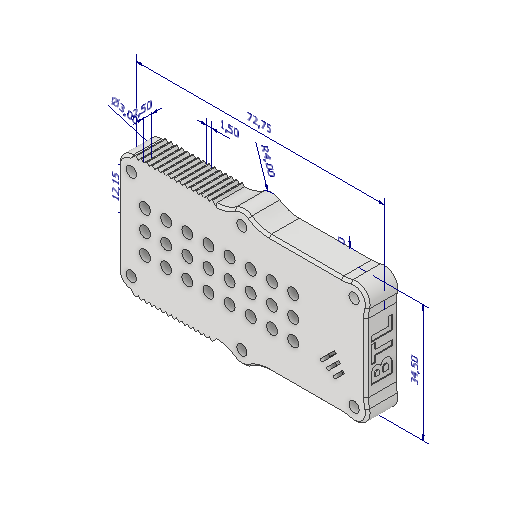
# Autodesk Inventor part: 3DP_PLA_Case_top_half
Saved by Autodesk Inventor 2025 (Build 290162010, 162A)
## iProperties
Created: 2018-09-08
Part Number: 3DP_PLA_Case_top_half
Material: ABS Plastic
Document SubType Name: Modeling
Designer: Andrzej
Density: 1.06 g/cm^3
Appearance: Smooth - White
Author: Andrzej
Autodesk Inventor part; units mm, degrees
ref_plane "YZ Plane" through (0, 0, 0) normal (1, 0, 0) x (0, 1, 0)
ref_plane "XZ Plane" through (0, 0, 0) normal (0, 1, 0) x (-1, 0, 0)
ref_plane "XY Plane" through (0, 0, 0) normal (0, 0, 1) x (1, 0, 0)
sketch "Sketch1" plane through (0, 0, 0) normal (0, 0, 1) x (1, 0, 0)
  line L0 (-37.547, 17.25) -> (35.203, 17.25)
  line L1 (35.203, 17.25) -> (35.203, -17.25)
  line L2 (35.203, -17.25) -> (-37.547, -17.25)
  line L3 (-37.547, -17.25) -> (-37.547, 17.25)
  line L4 (32.203, 14.25) -> (-34.547, 14.25)
  line L5 (-34.547, 14.25) -> (-34.547, -14.25)
  line L6 (-34.547, -14.25) -> (32.203, -14.25)
  line L7 (32.203, -14.25) -> (32.203, 14.25)
  point P0 (0, 0)
  dimension "d0" = 72.75
  dimension "d1" = 34.5
  dimension "d2" = 3
  dimension "d94" = 17.25
  constraints: 16 end point, 4 parallel, 2 perpendicular, 1 horizontal, 3 other
  measures "d0" distance of L1.end L2.end
  measures "d1" distance of L0.end L1.end
  measures "d2" distance between parallel lines of L0 L4
  measures "d94" distance from line of point (0, 0) L2
extrude "Extrusion1" add sketch "Sketch1" along normal blind 2.5 contours L0 L1 L2 L3 | L7 L6 L5 L4
extrude "Extrusion2" add sketch "Sketch1" against normal blind 6.3
fillet "Fillet1" radius 6 4 edges at (35.203, 17.25, -1.9) (32.203, 14.25, -3.15) (35.203, -17.25, -1.9) (32.203, -14.25, -3.15)
fillet "Fillet1" radius 4 4 edges at (-34.547, 14.25, -3.15) (-37.547, 17.25, -1.9) (-34.547, -14.25, -3.15) (-37.547, -17.25, -1.9)
sketch "Sketch2" plane through (0, 0, -6.3) normal (0, 0, -1) x (-1, 0, 0)
  line L0 (34.547, 10.25) -> (34.547, -10.25) projected
  arc A0 (30.547, -14.25) -> (34.547, -10.25) centre (30.547, -10.25) ccw projected
  line L1 (30.547, -14.25) -> (-26.203, -14.25) projected
  arc A1 (-32.203, -8.25) -> (-26.203, -14.25) centre (-26.203, -8.25) ccw projected
  line L2 (-32.203, -8.25) -> (-32.203, 8.25) projected
  arc A2 (-26.203, 14.25) -> (-32.203, 8.25) centre (-26.203, 8.25) ccw projected
  line L3 (-26.203, 14.25) -> (30.547, 14.25) projected
  arc A3 (34.547, 10.25) -> (30.547, 14.25) centre (30.547, 10.25) ccw projected
  arc A4 (33.547, -17.25) -> (37.547, -13.25) centre (33.547, -13.25) ccw projected
  line L4 (37.547, -13.25) -> (37.547, 13.25) projected
  arc A5 (37.547, 13.25) -> (33.547, 17.25) centre (33.547, 13.25) ccw projected
  line L5 (33.547, 17.25) -> (-29.203, 17.25) projected
  arc A6 (-29.203, 17.25) -> (-35.203, 11.25) centre (-29.203, 11.25) ccw projected
  line L6 (-35.203, 11.25) -> (-35.203, -11.25) projected
  arc A7 (-35.203, -11.25) -> (-29.203, -17.25) centre (-29.203, -11.25) ccw projected
  line L7 (-29.203, -17.25) -> (33.547, -17.25) projected
  circle A8 centre (33.547, 13.25) radius 4
  circle A9 centre (33.547, -13.25) radius 4
  circle A10 centre (1.172, -15.75) radius 4
  circle A11 centre (1.172, 15.75) radius 4
  circle A12 centre (-31.703, 13.75) radius 4
  circle A13 centre (-31.703, -13.75) radius 4
  point P0 (0, 0)
  dimension "d9" = 8
  dimension "d10" = 8
  dimension "d11" = 8
  dimension "d12" = 8
  dimension "d13" = 8
  dimension "d14" = 8
  dimension "d15" = 72.75
  dimension "d16" = 36.375
  dimension "d17" = 1.5
  dimension "d18" = 1.5
  dimension "d19" = 3.5
  dimension "d20" = 3.5
  dimension "d21" = 3.5
  constraints: 6 centre point, 2 coincident, 2 vertical alignment
  measures "d9" diameter of A8
  measures "d10" diameter of A9
  measures "d11" diameter of A10
  measures "d12" diameter of A11
  measures "d13" diameter of A12
  measures "d14" diameter of A13
  measures "d15" distance between parallel lines of L6 L4
  measures "d16" distance from line of L4 A10.centre
  measures "d17" distance from line of L5 A11.centre
  measures "d18" distance from line of L7 A10.centre
  measures "d19" distance from line of A13.centre L7
  measures "d20" distance from line of A13.centre L6
  measures "d21" distance from line of A12.centre L5
extrude "Extrusion3" add sketch "Sketch2" against normal up to surface (8.8 mm away) contours A3 L3 A8 A5 L0 | L0 A8 L3 A3 | A9 A4 L1 A0 L0 | L0 A0 L1 A9 | A11 L3 | L3 A11 L5 | A10 L7 L1 | L1 A10 | L5 A11 | A10 L7 | A12 A2 | A2 A12 A6 | A13 A7 A1 | A1 A13 | A6 A12 | A13 A7
hole "Hole1" at (31.703, -13.75, -6.3) at (-1.172, -15.75, -6.3) at (-33.547, -13.25, -6.3) at (-33.547, 13.25, -6.3) at (-1.172, 15.75, -6.3) at (31.703, 13.75, -6.3) direction (0, 0, 1) diameter 3 end through all both
sketch "Sketch3" plane through (-37.547, -13.25, 2.5) normal (-1, 0, 0) x (0, 0, 1)
  line L0 (0, 0) -> (-8.8, 0) projected
  line L1 (0, 26.5) -> (0, 0) projected
  line L2 (-8.8, 26.5) -> (0, 26.5) projected
  line L3 (-8.8, 0) -> (-8.8, 26.5) projected
  line L4 (-8.8, 5) -> (-8.8, 21.5) projected
  line L5 (-8.8, 19.325) -> (-6.1, 19.325)
  line L6 (-6.1, 19.325) -> (-6.1, 7.175)
  line L7 (-6.1, 7.175) -> (-8.8, 7.175)
  line L8 (-8.8, 7.175) -> (-8.8, 19.325)
  point P0 (-2.5, 13.25)
  dimension "d31" = 2.7
  dimension "d32" = 12.15
  dimension "d33" = 26.5
  dimension "d34" = 7.175
  constraints: 8 end point, 2 parallel, 1 horizontal, 1 perpendicular, 1 point on line
  measures "d31" distance of L6.end L7.end
  measures "d32" distance of L5.end L6.end
  measures "d33" distance between parallel lines of L0 L2
  measures "d34" distance between parallel lines of L2 L5
extrude "Extrusion4" cut sketch "Sketch3" against normal blind 8 contours L3 L5 L6 L7
sketch "Sketch4" plane through (0, 0, 0) normal (0, 0, -1) x (-1, 0, 0)
  arc A0 (34.547, -9.377) -> (29.674, -14.25) centre (33.547, -13.25) ccw projected
  line L0 (34.547, -9.377) -> (34.547, 9.377) projected
  arc A1 (29.674, 14.25) -> (34.547, 9.377) centre (33.547, 13.25) ccw projected
  line L1 (29.674, 14.25) -> (4.8801, 14.25) projected
  arc A2 (-2.5361, 14.25) -> (4.8801, 14.25) centre (1.172, 15.75) ccw projected
  line L2 (-2.5361, 14.25) -> (-26.203, 14.25) projected
  arc A3 (-26.203, 14.25) -> (-27.7148, 14.0564) centre (-26.203, 8.25) ccw projected
  arc A4 (-32.0095, 9.7618) -> (-27.7148, 14.0564) centre (-31.703, 13.75) ccw projected
  arc A5 (-32.0095, 9.7618) -> (-32.203, 8.25) centre (-26.203, 8.25) ccw projected
  line L3 (-32.203, 8.25) -> (-32.203, -8.25) projected
  arc A6 (-32.203, -8.25) -> (-32.0095, -9.7618) centre (-26.203, -8.25) ccw projected
  arc A7 (-27.7148, -14.0564) -> (-32.0095, -9.7618) centre (-31.703, -13.75) ccw projected
  arc A8 (-27.7148, -14.0564) -> (-26.203, -14.25) centre (-26.203, -8.25) ccw projected
  line L4 (-26.203, -14.25) -> (-2.5361, -14.25) projected
  arc A9 (4.8801, -14.25) -> (-2.5361, -14.25) centre (1.172, -15.75) ccw projected
  line L5 (4.8801, -14.25) -> (29.674, -14.25) projected
  line L6 (-32.203, 8.25) -> (-32.203, -8.25) projected
  line L7 (-32.203, 1) -> (-26.203, 1)
  line L8 (-26.203, 1) -> (-26.203, 5)
  line L9 (-26.203, 5) -> (-32.203, 5)
  line L10 (-32.203, 5) -> (-32.203, 1)
  line L11 (4.8801, -14.25) -> (29.674, -14.25) projected
  line L12 (17.047, -14.25) -> (12.047, -14.25)
  line L13 (12.047, -14.25) -> (12.047, -8.25)
  line L14 (12.047, -8.25) -> (17.047, -8.25)
  line L15 (17.047, -8.25) -> (17.047, -14.25)
  line L16 (-2.5361, -14.25) -> (-26.203, -14.25) projected
  line L17 (-13.953, -14.25) -> (-18.953, -14.25)
  line L18 (-18.953, -14.25) -> (-18.953, -8.25)
  line L19 (-18.953, -8.25) -> (-13.953, -8.25)
  line L20 (-13.953, -8.25) -> (-13.953, -14.25)
  line L21 (29.674, 14.25) -> (4.8801, 14.25) projected
  line L22 (15.547, 14.25) -> (10.547, 14.25)
  line L23 (10.547, 14.25) -> (10.547, 8.25)
  line L24 (10.547, 8.25) -> (15.547, 8.25)
  line L25 (15.547, 8.25) -> (15.547, 14.25)
  line L26 (-2.5361, 14.25) -> (-26.203, 14.25) projected
  line L27 (-8.953, 14.25) -> (-13.953, 14.25)
  line L28 (-13.953, 14.25) -> (-13.953, 8.25)
  line L29 (-13.953, 8.25) -> (-8.953, 8.25)
  line L30 (-8.953, 8.25) -> (-8.953, 14.25)
  point P0 (0, 0)
  dimension "d37" = 6
  dimension "d38" = 4
  dimension "d39" = 15.25
  dimension "d40" = 5
  dimension "d41" = 6
  dimension "d42" = 5
  dimension "d43" = 6
  dimension "d44" = 5
  dimension "d45" = 6
  dimension "d46" = 5
  dimension "d47" = 6
  dimension "d48" = 18.25
  dimension "d49" = 19
  dimension "d50" = 17.5
  dimension "d51" = 13.25
  constraints: 40 end point, 10 parallel, 5 horizontal, 5 perpendicular, 5 point on line
  measures "d37" distance of L9.end L8.end
  measures "d38" distance of L8.end L7.end
  measures "d39" distance between parallel lines of L7 L4
  measures "d40" distance of L13.end L14.end
  measures "d41" distance of L12.end L13.end
  measures "d42" distance of L18.end L19.end
  measures "d43" distance of L17.end L18.end
  measures "d44" distance of L24.end L23.end
  measures "d45" distance of L23.end L22.end
  measures "d46" distance of L29.end L28.end
  measures "d47" distance of L28.end L27.end
  measures "d48" distance between parallel lines of L3 L28
  measures "d49" distance between parallel lines of L0 L25
  measures "d50" distance between parallel lines of L0 L15
  measures "d51" distance between parallel lines of L3 L18
extrude "Extrusion5" add sketch "Sketch4" along normal blind 6.9 contours L5 L13 L14 L15 | L25 L24 L23 L1 | L4 L18 L19 L20 | L30 L29 L28 L2 | L3 L9 L8 L7
fillet "Fillet2" radius 2 20 edges at (-17.047, -14.25, -3.15) (-12.047, -14.25, -3.15) (13.953, -14.25, -3.15) (18.953, -14.25, -3.15) (32.203, 5, -3.15) (32.203, 1, -3.15) (8.953, 14.25, -3.15) (13.953, 14.25, -3.15) (-15.547, 14.25, -3.15) (-10.547, 14.25, -3.15) (-17.047, -8.25, -3.45) (-12.047, -8.25, -3.45) (-15.547, 8.25, -3.45) (-10.547, 8.25, -3.45) (8.953, 8.25, -3.45) (13.953, 8.25, -3.45) (13.953, -8.25, -3.45) (18.953, -8.25, -3.45) (26.203, 1, -3.45) (26.203, 5, -3.45)
chamfer "Chamfer1" distance 0.6 angle 45 5 edges at (-13.047, 14.25, -6.9) (11.453, 14.25, -6.9) (32.203, 3, -6.9) (16.453, -14.25, -6.9) (-14.547, -14.25, -6.9)
fillet "Fillet3" radius 10 8 edges at (-4.8801, 17.25, -1.9) (2.5361, 17.25, -1.9) (29.7258, 17.2272, -1.9) (35.1802, 11.7728, -1.9) (35.1802, -11.7728, -1.9) (29.7258, -17.2272, -1.9) (2.5361, -17.25, -1.9) (-4.8801, -17.25, -1.9)
sketch "Sketch5" plane through (0, 0, 0) normal (0, 0, -1) x (-1, 0, 0)
  arc A0 (10.547, 12.25) -> (8.547, 14.25) centre (8.547, 12.25) ccw projected
  line L0 (8.547, 14.25) -> (4.8801, 14.25) projected
  arc A1 (-2.5361, 14.25) -> (4.8801, 14.25) centre (1.172, 15.75) ccw projected
  line L1 (-2.5361, 14.25) -> (-6.953, 14.25) projected
  arc A2 (-6.953, 14.25) -> (-8.953, 12.25) centre (-6.953, 12.25) ccw projected
  line L2 (-8.953, 12.25) -> (-8.953, 10.25) projected
  arc A3 (-10.953, 8.25) -> (-8.953, 10.25) centre (-10.953, 10.25) ccw projected
  line L3 (-10.953, 8.25) -> (-11.953, 8.25) projected
  arc A4 (-13.953, 10.25) -> (-11.953, 8.25) centre (-11.953, 10.25) ccw projected
  line L4 (-13.953, 10.25) -> (-13.953, 12.25) projected
  arc A5 (-13.953, 12.25) -> (-15.953, 14.25) centre (-15.953, 12.25) ccw projected
  line L5 (-15.953, 14.25) -> (-26.203, 14.25) projected
  arc A6 (-26.203, 14.25) -> (-27.7148, 14.0564) centre (-26.203, 8.25) ccw projected
  arc A7 (-32.0095, 9.7618) -> (-27.7148, 14.0564) centre (-31.703, 13.75) ccw projected
  arc A8 (-32.0095, 9.7618) -> (-32.203, 8.25) centre (-26.203, 8.25) ccw projected
  line L6 (-32.203, 8.25) -> (-32.203, 7) projected
  arc A9 (-32.203, 7) -> (-30.203, 5) centre (-30.203, 7) ccw projected
  line L7 (-30.203, 5) -> (-28.203, 5) projected
  arc A10 (-28.203, 1) -> (-28.203, 5) centre (-28.203, 3) ccw projected
  line L8 (-28.203, 1) -> (-30.203, 1) projected
  arc A11 (-30.203, 1) -> (-32.203, -1) centre (-30.203, -1) ccw projected
  line L9 (-32.203, -1) -> (-32.203, -8.25) projected
  arc A12 (-32.203, -8.25) -> (-32.0095, -9.7618) centre (-26.203, -8.25) ccw projected
  arc A13 (-27.7148, -14.0564) -> (-32.0095, -9.7618) centre (-31.703, -13.75) ccw projected
  arc A14 (-27.7148, -14.0564) -> (-26.203, -14.25) centre (-26.203, -8.25) ccw projected
  line L10 (-26.203, -14.25) -> (-20.953, -14.25) projected
  arc A15 (-20.953, -14.25) -> (-18.953, -12.25) centre (-20.953, -12.25) ccw projected
  line L11 (-18.953, -12.25) -> (-18.953, -10.25) projected
  arc A16 (-16.953, -8.25) -> (-18.953, -10.25) centre (-16.953, -10.25) ccw projected
  line L12 (-16.953, -8.25) -> (-15.953, -8.25) projected
  arc A17 (-13.953, -10.25) -> (-15.953, -8.25) centre (-15.953, -10.25) ccw projected
  line L13 (-13.953, -10.25) -> (-13.953, -12.25) projected
  arc A18 (-13.953, -12.25) -> (-11.953, -14.25) centre (-11.953, -12.25) ccw projected
  line L14 (-11.953, -14.25) -> (-2.5361, -14.25) projected
  arc A19 (4.8801, -14.25) -> (-2.5361, -14.25) centre (1.172, -15.75) ccw projected
  line L15 (4.8801, -14.25) -> (10.047, -14.25) projected
  arc A20 (10.047, -14.25) -> (12.047, -12.25) centre (10.047, -12.25) ccw projected
  line L16 (12.047, -12.25) -> (12.047, -10.25) projected
  arc A21 (14.047, -8.25) -> (12.047, -10.25) centre (14.047, -10.25) ccw projected
  line L17 (14.047, -8.25) -> (15.047, -8.25) projected
  arc A22 (17.047, -10.25) -> (15.047, -8.25) centre (15.047, -10.25) ccw projected
  line L18 (17.047, -10.25) -> (17.047, -12.25) projected
  arc A23 (17.047, -12.25) -> (19.047, -14.25) centre (19.047, -12.25) ccw projected
  line L19 (19.047, -14.25) -> (29.674, -14.25) projected
  arc A24 (34.547, -9.377) -> (29.674, -14.25) centre (33.547, -13.25) ccw projected
  line L20 (34.547, -9.377) -> (34.547, 9.377) projected
  arc A25 (29.674, 14.25) -> (34.547, 9.377) centre (33.547, 13.25) ccw projected
  line L21 (29.674, 14.25) -> (17.547, 14.25) projected
  arc A26 (17.547, 14.25) -> (15.547, 12.25) centre (17.547, 12.25) ccw projected
  line L22 (15.547, 12.25) -> (15.547, 10.25) projected
  arc A27 (13.547, 8.25) -> (15.547, 10.25) centre (13.547, 10.25) ccw projected
  line L23 (13.547, 8.25) -> (12.547, 8.25) projected
  arc A28 (10.547, 10.25) -> (12.547, 8.25) centre (12.547, 10.25) ccw projected
  line L24 (10.547, 10.25) -> (10.547, 12.25) projected
  line L25 (-25.9217, -2.3862) -> (-21.6791, -6.6289)
  line L26 (-21.6791, -6.6289) -> (-22.2448, -7.1946)
  line L27 (-22.2448, -7.1946) -> (-26.4874, -2.9519)
  line L28 (-26.4874, -2.9519) -> (-25.9217, -2.3862)
  line L29 (-28.3259, -6.2046) -> (-25.4974, -9.033)
  line L30 (-25.4974, -9.033) -> (-26.0631, -9.5987)
  line L31 (-26.0631, -9.5987) -> (-28.8916, -6.7703)
  line L32 (-28.8916, -6.7703) -> (-28.3259, -6.2046)
  circle A29 centre (29.547, -6) radius 1.6
  circle A30 centre (23.347, -6) radius 1.6
  circle A31 centre (17.147, -6) radius 1.6
  circle A32 centre (10.947, -6) radius 1.6
  circle A33 centre (4.747, -6) radius 1.6
  circle A34 centre (-1.453, -6) radius 1.6
  circle A35 centre (-7.653, -6) radius 1.6
  circle A36 centre (-13.853, -6) radius 1.6
  circle A37 centre (29.547, 0) radius 1.6
  circle A38 centre (23.347, 0) radius 1.6
  circle A39 centre (17.147, 0) radius 1.6
  circle A40 centre (10.947, 0) radius 1.6
  circle A41 centre (4.747, 0) radius 1.6
  circle A42 centre (-1.453, 0) radius 1.6
  circle A43 centre (-7.653, 0) radius 1.6
  circle A44 centre (-13.853, 0) radius 1.6
  circle A45 centre (29.547, 6) radius 1.6
  circle A46 centre (23.347, 6) radius 1.6
  circle A47 centre (17.147, 6) radius 1.6
  circle A48 centre (10.947, 6) radius 1.6
  circle A49 centre (4.747, 6) radius 1.6
  circle A50 centre (-1.453, 6) radius 1.6
  circle A51 centre (-7.653, 6) radius 1.6
  circle A52 centre (-13.853, 6) radius 1.6
  line L33 (-27.1238, -4.2954) -> (-23.5883, -7.8309)
  line L34 (-23.5883, -7.8309) -> (-24.1539, -8.3966)
  line L35 (-24.1539, -8.3966) -> (-27.6895, -4.8611)
  line L36 (-27.6895, -4.8611) -> (-27.1238, -4.2954)
  point P0 (0, 0)
  dimension "d59" = 6
  dimension "d60" = 0.8
  dimension "d63" = 4
  dimension "d64" = 0.8
  dimension "d69" = 3.2
  dimension "d72" = 6.2
  dimension "d75" = 6
  dimension "d78" = 8.25
  dimension "d79" = 5
  dimension "d98" = 5
  dimension "d99" = 0.8
  dimension "d100" = 0.5
  dimension "d101" = 0.5
  dimension "d102" = 1.4
  dimension "d103" = 1.4
  constraints: 24 centre point, 24 end point, 6 parallel, 3 perpendicular, 1 horizontal, 1 vertical, 46 other
  measures "d59" distance of L26.end L27.end
  measures "d60" distance of L25.end L26.end
  measures "d63" distance of L31.start L32.start
  measures "d64" distance of L29.end L31.start
  measures "d69" diameter of A29
  measures "d72" distance of A29.centre A30.centre
  measures "d75" distance of A29.centre A37.centre
  measures "d78" distance from line of L19 A29.centre
  measures "d79" distance from line of L20 A29.centre
  measures "d98" distance of L34.end L35.end
  measures "d99" distance of L34.start L34.end
  measures "d100" distance between parallel lines of L36 L28
  measures "d101" distance between parallel lines of L34 L30
  measures "d102" distance between parallel lines of L27 L33
  measures "d103" distance between parallel lines of L29 L35
extrude "Extrusion6" cut sketch "Sketch5" against normal blind 8 contours L25 L26 L27 L28 | L29 L30 L31 L32 | A29 | A30 | A31 | A32 | A33 | A34 | A35 | A36 | A37 | A38 | A39 | A40 | A41 | A42 | A43 | A44 | A45 | A46 | A47 | A48 | A49 | A50 | A51 | A52 | L33 L34 L35 L36
fillet "Fillet4" radius 2 12 edges at (-34.547, -9.377, -3.15) (-29.674, -14.25, -3.15) (-4.8801, -14.25, -3.15) (2.5361, -14.25, -3.15) (27.7148, -14.0564, -3.15) (32.0095, -9.7618, -3.15) (32.0095, 9.7618, -3.15) (27.7148, 14.0564, -3.15) (2.5361, 14.25, -3.15) (-4.8801, 14.25, -3.15) (-34.547, 9.377, -3.15) (-29.674, 14.25, -3.15)
sketch "Sketch6" plane through (0, 0, -6.3) normal (0, 0, -1) x (-1, 0, 0)
  arc A0 (3.4532, 19.0357) -> (9.1563, 17.25) centre (9.1563, 27.25) ccw projected
  line L0 (9.1563, 17.25) -> (9.9063, 18)
  line L1 (9.1563, 17.25) -> (10.6563, 17.25) construction
  line L2 (10.6563, 17.25) -> (9.9063, 18)
  line L3 (10.6563, 17.25) -> (20.7753, 17.25) construction
  line L4 (9.1563, 17.25) -> (10.6563, 17.25)
  line L5 (33.547, 17.25) -> (9.1563, 17.25) projected
  point P0 (0, 0)
  dimension "d84" = 45
  dimension "d86" = 135
  dimension "d87" = 1.5
  constraints: 10 end point, 2 horizontal, 1 collinear
  measures "d84" angle of L1 L0
  measures "d86" angle of L3 L2
  measures "d87" distance of L0.start L1.end
extrude "Extrusion7" add sketch "Sketch6" against normal up to surface (8.8 mm away)
fillet "Fillet5" radius 0.2 1 edges at (-9.9063, 18, -1.9)
pattern_linear "Rectangular Pattern1" count 15 spacing 1.6 along (-1, 0, 0) of "Extrusion7", "Fillet5"
mirror "Mirror1" about plane through (0, 0, 0) normal (0, 1, 0) of "Extrusion7", "Fillet5", "Rectangular Pattern1"
chamfer "Chamfer2" distance 0.7 angle 45 20 edges at (-36.3754, -16.0784, 2.5) (-37.547, 0, 2.5) (-36.3754, 16.0784, 2.5) (-33.3017, 17.25, 2.5) (-33.3017, -17.25, 2.5) (17.4037, -17.25, 2.5) (29.3312, -17.3397, 2.5) (34.5315, -16.5784, 2.5) (35.2927, -11.3782, 2.5) (35.203, 0, 2.5) (35.2927, 11.3782, 2.5) (34.5315, 16.5784, 2.5) (29.3312, 17.3397, 2.5) (17.4037, 17.25, 2.5) (3.8243, 17.7069, 2.5) (-1.172, 19.75, 2.5) (-6.1683, 17.7069, 2.5) (3.8243, -17.7069, 2.5) (-1.172, -19.75, 2.5) (-6.1683, -17.7069, 2.5)
sketch "Sketch7" plane through (35.203, -10.0419, -6.3) normal (1, 0, 0) x (0, 0, -1)
  line L0 (-8.1, 0) -> (-8.1, 20.0838) projected
  line L1 (0, 0) -> (-8.1, 0) projected
  line L2 (0, 20.0838) -> (0, 0) projected
  line L3 (-8.1, 20.0838) -> (0, 20.0838) projected
  line L4 (-7.1997, 2.1091) -> (-7.1997, 8.241) construction
  line L5 (-7.1997, 8.241) -> (10.7816, 8.241) construction
  line L6 (10.7816, 8.241) -> (10.7816, 2.1091) construction
  line L7 (10.7816, 2.1091) -> (-7.1997, 2.1091) construction
  spline S0 degree 2 poles (-2.9682, 7.6159) (-2.5135, 7.6159) (-1.8264, 7.2699) (-1.599, 6.9832) knots 0 0 0 1 2 2 2
  spline S1 degree 2 poles (-1.599, 6.9832) (-1.3271, 6.6371) (-1.0997, 5.8166) (-1.0997, 5.1789) knots 0 0 0 1 2 2 2
  line L8 (-1.0997, 5.1789) -> (-1.0997, 2.7418)
  line L9 (-1.0997, 2.7418) -> (-7.1997, 2.7418)
  line L10 (-7.1997, 2.7418) -> (-7.1997, 4.8922)
  spline S2 degree 2 poles (-7.1997, 4.8922) (-7.1997, 5.5645) (-7.0959, 6.2565) (-6.9328, 6.5581) knots 0 0 0 1 2 2 2
  spline S3 degree 2 poles (-6.9328, 6.5581) (-6.7597, 6.8893) (-6.1665, 7.2106) (-5.781, 7.2106) knots 0 0 0 1 2 2 2
  spline S4 degree 2 poles (-5.781, 7.2106) (-5.3361, 7.2106) (-4.6391, 6.7657) (-4.4759, 6.3702) knots 0 0 0 1 2 2 2
  line L11 (-4.4759, 6.3702) -> (-4.4463, 6.3702)
  spline S5 degree 2 poles (-4.4463, 6.3702) (-4.3276, 6.9387) (-3.5911, 7.6159) (-2.9682, 7.6159) knots 0 0 0 1 2 2 2
  spline S6 degree 2 poles (-2.993, 6.0341) (-3.2797, 6.0341) (-3.601, 5.8067) (-3.685, 5.5793) knots 0 0 0 1 2 2 2
  spline S7 degree 2 poles (-3.685, 5.5793) (-3.7394, 5.4409) (-3.7493, 4.9515) (-3.7493, 4.5461) knots 0 0 0 1 2 2 2
  line L12 (-3.7493, 4.5461) -> (-3.7493, 4.2644)
  line L13 (-3.7493, 4.2644) -> (-2.2119, 4.2644)
  line L14 (-2.2119, 4.2644) -> (-2.2119, 4.3484)
  spline S8 degree 2 poles (-2.2119, 4.3484) (-2.2119, 4.9416) (-2.2268, 5.3964) (-2.3306, 5.6337) knots 0 0 0 1 2 2 2
  spline S9 degree 2 poles (-2.3306, 5.6337) (-2.4245, 5.8413) (-2.7705, 6.0341) (-2.993, 6.0341) knots 0 0 0 1 2 2 2
  spline S10 degree 2 poles (-5.4794, 5.6534) (-5.6277, 5.6534) (-5.9392, 5.5002) (-6.0084, 5.342) knots 0 0 0 1 2 2 2
  spline S11 degree 2 poles (-6.0084, 5.342) (-6.0776, 5.1937) (-6.0875, 4.7785) (-6.0875, 4.3682) knots 0 0 0 1 2 2 2
  line L15 (-6.0875, 4.3682) -> (-6.0875, 4.2644)
  line L16 (-6.0875, 4.2644) -> (-4.7923, 4.2644)
  line L17 (-4.7923, 4.2644) -> (-4.7923, 4.4572)
  spline S12 degree 2 poles (-4.7923, 4.4572) (-4.7923, 4.8477) (-4.8071, 5.164) (-4.8862, 5.3321) knots 0 0 0 1 2 2 2
  spline S13 degree 2 poles (-4.8862, 5.3321) (-4.9752, 5.515) (-5.2768, 5.6534) (-5.4794, 5.6534) knots 0 0 0 1 2 2 2
  line L18 (-1.0997, 9.6674) -> (-6.038, 9.6674)
  line L19 (-6.038, 9.6674) -> (-6.038, 7.8631)
  line L20 (-6.038, 7.8631) -> (-7.1997, 7.8631)
  line L21 (-7.1997, 7.8631) -> (-7.1997, 13.0041)
  line L22 (-7.1997, 13.0041) -> (-6.038, 13.0041)
  line L23 (-6.038, 13.0041) -> (-6.038, 11.1998)
  line L24 (-6.038, 11.1998) -> (-1.0997, 11.1998)
  line L25 (-1.0997, 11.1998) -> (-1.0997, 9.6674)
  line L26 (-1.0997, 17.7002) -> (-1.0997, 13.6319)
  line L27 (-1.0997, 13.6319) -> (-7.1997, 13.6319)
  line L28 (-7.1997, 13.6319) -> (-7.1997, 15.1643)
  line L29 (-7.1997, 15.1643) -> (-2.2614, 15.1643)
  line L30 (-2.2614, 15.1643) -> (-2.2614, 17.7002)
  line L31 (-2.2614, 17.7002) -> (-1.0997, 17.7002)
  point P0 (-6.3, 10.0419)
  constraints: 2 other
extrude "Extrusion8" cut sketch "Sketch7" against normal blind 0.25 contours S0 S1 L8 L9 L10 S2 S3 S4 L11 S5 | L18 L19 L20 L21 L22 L23 L24 L25 | L26 L27 L28 L29 L30 L31
sketch "Sketch8" plane through (6.8124, -17.25, -6.3) normal (0, -1, 0) x (1, 0, 0)
  line L0 (0, 8.1) -> (21.1825, 8.1) projected
  line L1 (0, 0) -> (0, 8.1) projected
  line L2 (21.1825, 0) -> (0, 0) projected
  line L3 (21.1825, 8.1) -> (21.1825, 0) projected
  line L4 (2.5381, 7.0964) -> (22.7439, 7.0964) construction
  line L5 (22.7439, 7.0964) -> (22.7439, -4.5758) construction
  line L6 (22.7439, -4.5758) -> (2.5381, -4.5758) construction
  line L7 (2.5381, -4.5758) -> (2.5381, 7.0964) construction
  line L8 (8.8062, 0.9964) -> (6.9426, 0.9964)
  line L9 (6.9426, 0.9964) -> (5.2471, 3.2357)
  line L10 (5.2471, 3.2357) -> (4.6934, 3.2357)
  line L11 (4.6934, 3.2357) -> (4.6934, 0.9964)
  line L12 (4.6934, 0.9964) -> (3.1709, 0.9964)
  line L13 (3.1709, 0.9964) -> (3.1709, 7.0964)
  line L14 (3.1709, 7.0964) -> (5.6227, 7.0964)
  spline S0 degree 2 poles (5.6227, 7.0964) (6.1319, 7.0964) (6.8833, 6.9679) (7.2046, 6.7701) knots 0 0 0 1 2 2 2
  spline S1 degree 2 poles (7.2046, 6.7701) (7.5308, 6.5625) (7.9164, 5.9149) (7.9164, 5.4206) knots 0 0 0 1 2 2 2
  spline S2 degree 2 poles (7.9164, 5.4206) (7.9164, 4.7236) (7.2837, 3.8487) (6.7548, 3.5916) knots 0 0 0 1 2 2 2
  line L15 (6.7548, 3.5916) -> (8.8062, 0.9964)
  spline S3 degree 2 poles (6.3445, 5.2278) (6.3445, 5.4602) (6.1665, 5.7914) (5.9638, 5.8803) knots 0 0 0 1 2 2 2
  spline S4 degree 2 poles (5.9638, 5.8803) (5.8205, 5.9397) (5.4695, 5.9743) (5.2075, 5.9743) knots 0 0 0 1 2 2 2
  line L16 (5.2075, 5.9743) -> (4.6934, 5.9743)
  line L17 (4.6934, 5.9743) -> (4.6934, 4.3331)
  line L18 (4.6934, 4.3331) -> (5.1334, 4.3331)
  spline S5 degree 2 poles (5.1334, 4.3331) (5.4497, 4.3331) (5.8996, 4.4122) (6.0528, 4.5358) knots 0 0 0 1 2 2 2
  spline S6 degree 2 poles (6.0528, 4.5358) (6.2011, 4.6544) (6.3445, 4.9708) (6.3445, 5.2278) knots 0 0 0 1 2 2 2
  line L19 (10.4325, 0.9964) -> (10.4325, 5.9347)
  line L20 (10.4325, 5.9347) -> (8.6283, 5.9347)
  line L21 (8.6283, 5.9347) -> (8.6283, 7.0964)
  line L22 (8.6283, 7.0964) -> (13.7693, 7.0964)
  line L23 (13.7693, 7.0964) -> (13.7693, 5.9347)
  line L24 (13.7693, 5.9347) -> (11.965, 5.9347)
  line L25 (11.965, 5.9347) -> (11.965, 0.9964)
  line L26 (11.965, 0.9964) -> (10.4325, 0.9964)
  line L27 (18.4654, 0.9964) -> (14.3971, 0.9964)
  line L28 (14.3971, 0.9964) -> (14.3971, 7.0964)
  line L29 (14.3971, 7.0964) -> (15.9295, 7.0964)
  line L30 (15.9295, 7.0964) -> (15.9295, 2.1581)
  line L31 (15.9295, 2.1581) -> (18.4654, 2.1581)
  line L32 (18.4654, 2.1581) -> (18.4654, 0.9964)
  point P0 (-6.8124, 6.3)
  constraints: 2 other
extrude "Extrusion9" cut sketch "Sketch8" against normal blind 0.25 contours L8 L9 L10 L11 L12 L13 L14 S0 S1 S2 L15 | L19 L20 L21 L22 L23 L24 L25 L26 | L27 L28 L29 L30 L31 L32
sketch "Sketch9" plane through (0, 0, -6.9) normal (0, 0, -1) x (-1, 0, 0)
  arc A0 (32.1649, -17.8586) -> (32.4478, -17.8586) centre (32.3063, -17.7172) ccw projected
  line L0 (33.0563, -17.25) -> (32.4478, -17.8586) projected
  line L1 (33.0563, -17.25) -> (33.547, -17.25) projected
  arc A1 (33.547, -17.25) -> (37.547, -13.25) centre (33.547, -13.25) ccw projected
  line L2 (37.547, -13.25) -> (37.547, -6.075) projected
  line L3 (37.547, -6.075) -> (34.547, -6.075) projected
  line L4 (34.547, -6.075) -> (34.547, -7.3339) projected
  arc A2 (32.8803, -9.3059) -> (34.547, -7.3339) centre (32.547, -7.3339) ccw projected
  arc A3 (32.8803, -9.3059) -> (29.6029, -12.5833) centre (33.547, -13.25) ccw projected
  arc A4 (27.6309, -14.25) -> (29.6029, -12.5833) centre (27.6309, -12.25) ccw projected
  line L5 (27.6309, -14.25) -> (19.047, -14.25) projected
  arc A5 (17.047, -12.25) -> (19.047, -14.25) centre (19.047, -12.25) ccw projected
  line L6 (17.047, -14.25) -> (17.047, -12.25) projected
  line L7 (17.047, -14.25) -> (12.047, -14.25) projected
  line L8 (12.047, -12.25) -> (12.047, -14.25) projected
  arc A6 (10.047, -14.25) -> (12.047, -12.25) centre (10.047, -12.25) ccw projected
  line L9 (10.047, -14.25) -> (6.0454, -14.25) projected
  arc A7 (4.4209, -13.4167) -> (6.0454, -14.25) centre (6.0454, -12.25) ccw projected
  arc A8 (4.4209, -13.4167) -> (-2.077, -13.4167) centre (1.172, -15.75) ccw projected
  arc A9 (-3.7014, -14.25) -> (-2.077, -13.4167) centre (-3.7014, -12.25) ccw projected
  line L10 (-3.7014, -14.25) -> (-11.953, -14.25) projected
  arc A10 (-13.953, -12.25) -> (-11.953, -14.25) centre (-11.953, -12.25) ccw projected
  line L11 (-13.953, -14.25) -> (-13.953, -12.25) projected
  line L12 (-13.953, -14.25) -> (-18.953, -14.25) projected
  line L13 (-18.953, -12.25) -> (-18.953, -14.25) projected
  arc A11 (-20.953, -14.25) -> (-18.953, -12.25) centre (-20.953, -12.25) ccw projected
  line L14 (-20.953, -14.25) -> (-25.8935, -14.25) projected
  arc A12 (-27.83, -12.75) -> (-25.8935, -14.25) centre (-25.8935, -12.25) ccw projected
  arc A13 (-27.83, -12.75) -> (-30.703, -9.877) centre (-31.703, -13.75) ccw projected
  arc A14 (-32.203, -7.9405) -> (-30.703, -9.877) centre (-30.203, -7.9405) ccw projected
  line L15 (-32.203, -7.9405) -> (-32.203, -1) projected
  arc A15 (-30.203, 1) -> (-32.203, -1) centre (-30.203, -1) ccw projected
  line L16 (-32.203, 1) -> (-30.203, 1) projected
  line L17 (-32.203, 1) -> (-32.203, 5) projected
  line L18 (-30.203, 5) -> (-32.203, 5) projected
  arc A16 (-32.203, 7) -> (-30.203, 5) centre (-30.203, 7) ccw projected
  line L19 (-32.203, 7) -> (-32.203, 7.9405) projected
  arc A17 (-30.703, 9.877) -> (-32.203, 7.9405) centre (-30.203, 7.9405) ccw projected
  arc A18 (-30.703, 9.877) -> (-27.83, 12.75) centre (-31.703, 13.75) ccw projected
  arc A19 (-25.8935, 14.25) -> (-27.83, 12.75) centre (-25.8935, 12.25) ccw projected
  line L20 (-25.8935, 14.25) -> (-15.953, 14.25) projected
  arc A20 (-13.953, 12.25) -> (-15.953, 14.25) centre (-15.953, 12.25) ccw projected
  line L21 (-13.953, 14.25) -> (-13.953, 12.25) projected
  line L22 (-13.953, 14.25) -> (-8.953, 14.25) projected
  line L23 (-8.953, 12.25) -> (-8.953, 14.25) projected
  arc A21 (-6.953, 14.25) -> (-8.953, 12.25) centre (-6.953, 12.25) ccw projected
  line L24 (-6.953, 14.25) -> (-3.7014, 14.25) projected
  arc A22 (-2.077, 13.4167) -> (-3.7014, 14.25) centre (-3.7014, 12.25) ccw projected
  arc A23 (-2.077, 13.4167) -> (4.4209, 13.4167) centre (1.172, 15.75) ccw projected
  arc A24 (6.0454, 14.25) -> (4.4209, 13.4167) centre (6.0454, 12.25) ccw projected
  line L25 (6.0454, 14.25) -> (8.547, 14.25) projected
  arc A25 (10.547, 12.25) -> (8.547, 14.25) centre (8.547, 12.25) ccw projected
  line L26 (10.547, 14.25) -> (10.547, 12.25) projected
  line L27 (10.547, 14.25) -> (15.547, 14.25) projected
  line L28 (15.547, 12.25) -> (15.547, 14.25) projected
  arc A26 (17.547, 14.25) -> (15.547, 12.25) centre (17.547, 12.25) ccw projected
  line L29 (17.547, 14.25) -> (27.6309, 14.25) projected
  arc A27 (29.6029, 12.5833) -> (27.6309, 14.25) centre (27.6309, 12.25) ccw projected
  arc A28 (29.6029, 12.5833) -> (32.8803, 9.3059) centre (33.547, 13.25) ccw projected
  arc A29 (34.547, 7.3339) -> (32.8803, 9.3059) centre (32.547, 7.3339) ccw projected
  line L30 (34.547, 7.3339) -> (34.547, 6.075) projected
  line L31 (34.547, 6.075) -> (37.547, 6.075) projected
  line L32 (37.547, 6.075) -> (37.547, 13.25) projected
  arc A30 (37.547, 13.25) -> (33.547, 17.25) centre (33.547, 13.25) ccw projected
  line L33 (33.547, 17.25) -> (33.0563, 17.25) projected
  line L34 (33.0563, 17.25) -> (32.4478, 17.8586) projected
  arc A31 (32.4478, 17.8586) -> (32.1649, 17.8586) centre (32.3063, 17.7172) ccw projected
  line L35 (32.1649, 17.8586) -> (31.5563, 17.25) projected
  line L36 (31.5563, 17.25) -> (31.4563, 17.25) projected
  line L37 (31.4563, 17.25) -> (30.8478, 17.8586) projected
  arc A32 (30.8478, 17.8586) -> (30.5649, 17.8586) centre (30.7063, 17.7172) ccw projected
  line L38 (30.5649, 17.8586) -> (29.9563, 17.25) projected
  line L39 (29.9563, 17.25) -> (29.8563, 17.25) projected
  line L40 (29.8563, 17.25) -> (29.2478, 17.8586) projected
  arc A33 (29.2478, 17.8586) -> (28.9649, 17.8586) centre (29.1063, 17.7172) ccw projected
  line L41 (28.9649, 17.8586) -> (28.3563, 17.25) projected
  line L42 (28.3563, 17.25) -> (28.2563, 17.25) projected
  line L43 (28.2563, 17.25) -> (27.6478, 17.8586) projected
  arc A34 (27.6478, 17.8586) -> (27.3649, 17.8586) centre (27.5063, 17.7172) ccw projected
  line L44 (27.3649, 17.8586) -> (26.7563, 17.25) projected
  line L45 (26.7563, 17.25) -> (26.6563, 17.25) projected
  line L46 (26.6563, 17.25) -> (26.0478, 17.8586) projected
  arc A35 (26.0478, 17.8586) -> (25.7649, 17.8586) centre (25.9063, 17.7172) ccw projected
  line L47 (25.7649, 17.8586) -> (25.1563, 17.25) projected
  line L48 (25.1563, 17.25) -> (25.0563, 17.25) projected
  line L49 (25.0563, 17.25) -> (24.4478, 17.8586) projected
  arc A36 (24.4478, 17.8586) -> (24.1649, 17.8586) centre (24.3063, 17.7172) ccw projected
  line L50 (24.1649, 17.8586) -> (23.5563, 17.25) projected
  line L51 (23.5563, 17.25) -> (23.4563, 17.25) projected
  line L52 (23.4563, 17.25) -> (22.8478, 17.8586) projected
  arc A37 (22.8478, 17.8586) -> (22.5649, 17.8586) centre (22.7063, 17.7172) ccw projected
  line L53 (22.5649, 17.8586) -> (21.9563, 17.25) projected
  line L54 (21.9563, 17.25) -> (21.8563, 17.25) projected
  line L55 (21.8563, 17.25) -> (21.2478, 17.8586) projected
  arc A38 (21.2478, 17.8586) -> (20.9649, 17.8586) centre (21.1063, 17.7172) ccw projected
  line L56 (20.9649, 17.8586) -> (20.3563, 17.25) projected
  line L57 (20.3563, 17.25) -> (20.2563, 17.25) projected
  line L58 (20.2563, 17.25) -> (19.6478, 17.8586) projected
  arc A39 (19.6478, 17.8586) -> (19.3649, 17.8586) centre (19.5063, 17.7172) ccw projected
  line L59 (19.3649, 17.8586) -> (18.7563, 17.25) projected
  line L60 (18.7563, 17.25) -> (18.6563, 17.25) projected
  line L61 (18.6563, 17.25) -> (18.0478, 17.8586) projected
  arc A40 (18.0478, 17.8586) -> (17.7649, 17.8586) centre (17.9063, 17.7172) ccw projected
  line L62 (17.7649, 17.8586) -> (17.1563, 17.25) projected
  line L63 (17.1563, 17.25) -> (17.0563, 17.25) projected
  line L64 (17.0563, 17.25) -> (16.4478, 17.8586) projected
  arc A41 (16.4478, 17.8586) -> (16.1649, 17.8586) centre (16.3063, 17.7172) ccw projected
  line L65 (16.1649, 17.8586) -> (15.5563, 17.25) projected
  line L66 (15.5563, 17.25) -> (15.4563, 17.25) projected
  line L67 (15.4563, 17.25) -> (14.8478, 17.8586) projected
  arc A42 (14.8478, 17.8586) -> (14.5649, 17.8586) centre (14.7063, 17.7172) ccw projected
  line L68 (14.5649, 17.8586) -> (13.9563, 17.25) projected
  line L69 (13.9563, 17.25) -> (13.8563, 17.25) projected
  line L70 (13.8563, 17.25) -> (13.2478, 17.8586) projected
  arc A43 (13.2478, 17.8586) -> (12.9649, 17.8586) centre (13.1063, 17.7172) ccw projected
  line L71 (12.9649, 17.8586) -> (12.3563, 17.25) projected
  line L72 (12.3563, 17.25) -> (12.2563, 17.25) projected
  line L73 (12.2563, 17.25) -> (11.6478, 17.8586) projected
  arc A44 (11.6478, 17.8586) -> (11.3649, 17.8586) centre (11.5063, 17.7172) ccw projected
  line L74 (11.3649, 17.8586) -> (10.7563, 17.25) projected
  line L75 (10.7563, 17.25) -> (10.6563, 17.25) projected
  line L76 (10.6563, 17.25) -> (10.0478, 17.8586) projected
  arc A45 (10.0478, 17.8586) -> (9.7649, 17.8586) centre (9.9063, 17.7172) ccw projected
  line L77 (9.7649, 17.8586) -> (9.1563, 17.25) projected
  arc A46 (3.4532, 19.0357) -> (9.1563, 17.25) centre (9.1563, 27.25) ccw projected
  arc A47 (3.4532, 19.0357) -> (-1.1093, 19.0357) centre (1.172, 15.75) ccw projected
  arc A48 (-6.8124, 17.25) -> (-1.1093, 19.0357) centre (-6.8124, 27.25) ccw projected
  line L78 (-6.8124, 17.25) -> (-27.9949, 17.25) projected
  arc A49 (-30.6436, 17.6071) -> (-27.9949, 17.25) centre (-27.9949, 27.25) ccw projected
  arc A50 (-30.6436, 17.6071) -> (-35.5602, 12.6905) centre (-31.703, 13.75) ccw projected
  arc A51 (-35.203, 10.0419) -> (-35.5602, 12.6905) centre (-45.203, 10.0419) ccw projected
  line L79 (-35.203, 10.0419) -> (-35.203, -10.0419) projected
  arc A52 (-35.5602, -12.6905) -> (-35.203, -10.0419) centre (-45.203, -10.0419) ccw projected
  arc A53 (-35.5602, -12.6905) -> (-30.6436, -17.6071) centre (-31.703, -13.75) ccw projected
  arc A54 (-27.9949, -17.25) -> (-30.6436, -17.6071) centre (-27.9949, -27.25) ccw projected
  line L80 (-27.9949, -17.25) -> (-6.8124, -17.25) projected
  arc A55 (-1.1093, -19.0357) -> (-6.8124, -17.25) centre (-6.8124, -27.25) ccw projected
  arc A56 (-1.1093, -19.0357) -> (3.4532, -19.0357) centre (1.172, -15.75) ccw projected
  arc A57 (9.1563, -17.25) -> (3.4532, -19.0357) centre (9.1563, -27.25) ccw projected
  line L81 (9.7649, -17.8586) -> (9.1563, -17.25) projected
  arc A58 (9.7649, -17.8586) -> (10.0478, -17.8586) centre (9.9063, -17.7172) ccw projected
  line L82 (10.6563, -17.25) -> (10.0478, -17.8586) projected
  line L83 (10.6563, -17.25) -> (10.7563, -17.25) projected
  line L84 (11.3649, -17.8586) -> (10.7563, -17.25) projected
  arc A59 (11.3649, -17.8586) -> (11.6478, -17.8586) centre (11.5063, -17.7172) ccw projected
  line L85 (12.2563, -17.25) -> (11.6478, -17.8586) projected
  line L86 (12.2563, -17.25) -> (12.3563, -17.25) projected
  line L87 (12.9649, -17.8586) -> (12.3563, -17.25) projected
  arc A60 (12.9649, -17.8586) -> (13.2478, -17.8586) centre (13.1063, -17.7172) ccw projected
  line L88 (13.8563, -17.25) -> (13.2478, -17.8586) projected
  line L89 (13.8563, -17.25) -> (13.9563, -17.25) projected
  line L90 (14.5649, -17.8586) -> (13.9563, -17.25) projected
  arc A61 (14.5649, -17.8586) -> (14.8478, -17.8586) centre (14.7063, -17.7172) ccw projected
  line L91 (15.4563, -17.25) -> (14.8478, -17.8586) projected
  line L92 (15.4563, -17.25) -> (15.5563, -17.25) projected
  line L93 (16.1649, -17.8586) -> (15.5563, -17.25) projected
  arc A62 (16.1649, -17.8586) -> (16.4478, -17.8586) centre (16.3063, -17.7172) ccw projected
  line L94 (17.0563, -17.25) -> (16.4478, -17.8586) projected
  line L95 (17.0563, -17.25) -> (17.1563, -17.25) projected
  line L96 (17.7649, -17.8586) -> (17.1563, -17.25) projected
  arc A63 (17.7649, -17.8586) -> (18.0478, -17.8586) centre (17.9063, -17.7172) ccw projected
  line L97 (18.6563, -17.25) -> (18.0478, -17.8586) projected
  line L98 (18.6563, -17.25) -> (18.7563, -17.25) projected
  line L99 (19.3649, -17.8586) -> (18.7563, -17.25) projected
  arc A64 (19.3649, -17.8586) -> (19.6478, -17.8586) centre (19.5063, -17.7172) ccw projected
  line L100 (20.2563, -17.25) -> (19.6478, -17.8586) projected
  line L101 (20.2563, -17.25) -> (20.3563, -17.25) projected
  line L102 (20.9649, -17.8586) -> (20.3563, -17.25) projected
  arc A65 (20.9649, -17.8586) -> (21.2478, -17.8586) centre (21.1063, -17.7172) ccw projected
  line L103 (21.8563, -17.25) -> (21.2478, -17.8586) projected
  line L104 (21.8563, -17.25) -> (21.9563, -17.25) projected
  line L105 (22.5649, -17.8586) -> (21.9563, -17.25) projected
  arc A66 (22.5649, -17.8586) -> (22.8478, -17.8586) centre (22.7063, -17.7172) ccw projected
  line L106 (23.4563, -17.25) -> (22.8478, -17.8586) projected
  line L107 (23.4563, -17.25) -> (23.5563, -17.25) projected
  line L108 (24.1649, -17.8586) -> (23.5563, -17.25) projected
  arc A67 (24.1649, -17.8586) -> (24.4478, -17.8586) centre (24.3063, -17.7172) ccw projected
  line L109 (25.0563, -17.25) -> (24.4478, -17.8586) projected
  line L110 (25.0563, -17.25) -> (25.1563, -17.25) projected
  line L111 (25.7649, -17.8586) -> (25.1563, -17.25) projected
  arc A68 (25.7649, -17.8586) -> (26.0478, -17.8586) centre (25.9063, -17.7172) ccw projected
  line L112 (26.6563, -17.25) -> (26.0478, -17.8586) projected
  line L113 (26.6563, -17.25) -> (26.7563, -17.25) projected
  line L114 (27.3649, -17.8586) -> (26.7563, -17.25) projected
  arc A69 (27.3649, -17.8586) -> (27.6478, -17.8586) centre (27.5063, -17.7172) ccw projected
  line L115 (28.2563, -17.25) -> (27.6478, -17.8586) projected
  line L116 (28.2563, -17.25) -> (28.3563, -17.25) projected
  line L117 (28.9649, -17.8586) -> (28.3563, -17.25) projected
  arc A70 (28.9649, -17.8586) -> (29.2478, -17.8586) centre (29.1063, -17.7172) ccw projected
  line L118 (29.8563, -17.25) -> (29.2478, -17.8586) projected
  line L119 (29.8563, -17.25) -> (29.9563, -17.25) projected
  line L120 (30.5649, -17.8586) -> (29.9563, -17.25) projected
  arc A71 (30.5649, -17.8586) -> (30.8478, -17.8586) centre (30.7063, -17.7172) ccw projected
  line L121 (31.4563, -17.25) -> (30.8478, -17.8586) projected
  line L122 (31.4563, -17.25) -> (31.5563, -17.25) projected
  line L123 (32.1649, -17.8586) -> (31.5563, -17.25) projected
  circle A72 centre (-31.703, 13.75) radius 1.5 projected
  circle A73 centre (33.547, 13.25) radius 1.5 projected
  circle A74 centre (1.172, -15.75) radius 1.5 projected
  circle A75 centre (-31.703, -13.75) radius 1.5 projected
  circle A76 centre (33.547, -13.25) radius 1.5 projected
  circle A77 centre (1.172, 15.75) radius 1.5 projected
  line L124 (-32.203, -7.9405) -> (-32.203, -1) projected
  line L125 (-32.203, -1) -> (-25.2956, -1)
  line L126 (-25.2956, -1) -> (-25.2956, 7.6165)
  line L127 (-25.2956, 7.6165) -> (-32.203, 7.6165)
  line L128 (-32.203, 7.6165) -> (-32.203, -1)
  point P0 (0, 0)
  constraints: 8 end point, 2 parallel, 1 horizontal, 1 perpendicular
extrude "Extrusion10" cut sketch "Sketch9" against normal up to surface (6.9 mm away) contours L128 L16 A15 | A15 L16 L17 L18 A16 L19 L127 L126 L125 | L128 A16 L18
equation "\"d94\" = 0.5 * d1"
equation "\"d16\" = 0.5 * d15"
equation "\"d34\" = -0.5 * d32 + 0.5 * d33"
body "Solid1"
